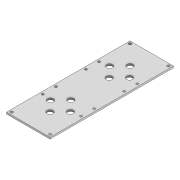
# Autodesk Inventor part: Cover
Saved by Autodesk Inventor 2022 (Build 260153000, 153)
## iProperties
Created: 2021-11-16
Part Number: Cover
Material: Generic
Document SubType Name: Modeling
Designer: Vking
Density: 1 g/cm^3
Appearance: Default
Author: Vking
Autodesk Inventor part; units mm, degrees
ref_plane "YZ Plane" through (0, 0, 0) normal (1, 0, 0) x (0, 1, 0)
ref_plane "XZ Plane" through (0, 0, 0) normal (0, 1, 0) x (-1, 0, 0)
ref_plane "XY Plane" through (0, 0, 0) normal (0, 0, 1) x (1, 0, 0)
sketch "Sketch1" plane through (0, 0, 0) normal (0, 1, 0) x (-1, 0, 0)
  line L0 (28.7334, 91.142) -> (-21.2666, 91.142)
  line L1 (-21.2666, 91.142) -> (-21.2666, -78.858)
  line L2 (-21.2666, -78.858) -> (28.7334, -78.858)
  line L3 (28.7334, -78.858) -> (28.7334, 91.142)
  line L4 (36.3534, 98.762) -> (-28.8866, 98.762)
  line L5 (-28.8866, 98.762) -> (-28.8866, -86.478)
  line L6 (-28.8866, -86.478) -> (36.3534, -86.478)
  line L7 (36.3534, -86.478) -> (36.3534, 98.762)
  circle A0 centre (3.7334, 66.142) radius 4.5
  circle A1 centre (18.7334, 50.521) radius 4.5
  circle A2 centre (3.7334, 34.892) radius 4.5
  circle A3 centre (-11.2666, 50.521) radius 4.5
  circle A4 centre (3.7334, -22.616) radius 4.5
  circle A5 centre (18.7334, -38.237) radius 4.5
  circle A6 centre (-11.2666, -38.237) radius 4.5
  circle A7 centre (3.7334, -53.858) radius 4.5
  circle A8 centre (32.5434, 94.952) radius 2
  circle A9 centre (-25.0766, 94.952) radius 2
  circle A10 centre (-25.0766, -82.668) radius 2
  circle A11 centre (32.5434, -82.668) radius 2
  circle A12 centre (32.3534, -16.3569) radius 1.695
  circle A13 centre (32.3656, 28.6431) radius 1.695
  circle A14 centre (32.3534, -36.0528) radius 1.6891
  circle A15 centre (32.3656, 48.339) radius 1.6891
  line L8 (3.7397, -95.1843) -> (3.7397, 116.3603) construction
  circle A16 centre (-24.874, -16.3569) radius 1.695
  circle A17 centre (-24.8862, 28.6431) radius 1.695
  circle A18 centre (-24.874, -36.0528) radius 1.6891
  circle A19 centre (-24.8862, 48.339) radius 1.6891
  point P0 (0, 0)
  dimension "d0" = 170
  dimension "d1" = 7.62
  dimension "d2" = 9
  dimension "d4" = 10
  dimension "d5" = 10
  dimension "d6" = 9
  dimension "d7" = 25
  dimension "d8" = 25
  dimension "d9" = 50
  dimension "d10" = 10
  dimension "d11" = 10
  dimension "d12" = 25
  dimension "d13" = 25
  dimension "d14" = 31.25
  dimension "d15" = 25
  dimension "d16" = 9
  dimension "d17" = 9
  dimension "d18" = 15.621
  dimension "d19" = 0
  dimension "d21" = 25
  dimension "d22" = 31.242
  dimension "d23" = 15.621
  dimension "d24" = 9
  dimension "d25" = 9
  dimension "d26" = 9
  dimension "d27" = 9
  dimension "d29" = 15.621
  dimension "d34" = 3.81
  dimension "d35" = 3.81
  dimension "d36" = 4
  dimension "d37" = 3.81
  dimension "d38" = 3.81
  dimension "d39" = 4
  dimension "d40" = 3.81
  dimension "d41" = 3.81
  dimension "d42" = 4
  dimension "d43" = 3.81
  dimension "d44" = 3.81
  dimension "d45" = 4
  dimension "d49" = 4
  dimension "d50" = 45
  dimension "d51" = 70.1211
  dimension "d52" = 3.9878
  dimension "d53" = 3.39
  dimension "d54" = 3.39
  dimension "d55" = 0
  dimension "d56" = 3.3782
  dimension "d57" = 0
  dimension "d58" = 23.08
  dimension "d59" = 23.08
  dimension "d60" = 32.6263
  dimension "d61" = 3.3782
  dimension "d62" = 4.0004
  constraints: 20 centre point, 18 end point, 4 parallel, 4 symmetric about line, 2 perpendicular, 1 horizontal, 1 vertical, 7 other
  measures "d0" distance of L2.end L0.start
  measures "d1" distance between parallel lines of L3 L7
  measures "d2" diameter of A1
  measures "d4" distance from line of A1.centre L3
  measures "d5" distance from line of L1 A3.centre
  measures "d6" diameter of A3
  measures "d7" distance from line of L1 A2.centre
  measures "d8" distance from line of L1 A0.centre
  measures "d9" distance of L1.end L2.end
  measures "d10" distance from line of L1 A6.centre
  measures "d11" distance from line of A5.centre L3
  measures "d12" distance from line of L1 A4.centre
  measures "d13" distance from line of L1 A7.centre
  measures "d14" distance of A2.centre A0.centre
  measures "d15" distance from line of L0 A0.centre
  measures "d16" diameter of A0
  measures "d17" diameter of A2
  measures "d18" vertical distance of A3.centre A0.centre
  measures "d19" vertical distance of A3.centre A1.centre
  measures "d21" distance from line of L2 A7.centre
  measures "d22" distance of A4.centre A7.centre
  measures "d23" vertical distance of A6.centre A4.centre
  measures "d24" diameter of A4
  measures "d25" diameter of A6
  measures "d26" diameter of A7
  measures "d27" diameter of A5
  measures "d29" vertical distance of A7.centre A5.centre
  measures "d34" distance from line of L6 A11.centre
  measures "d35" distance from line of A11.centre L7
  measures "d36" diameter of A11
  measures "d37" distance from line of L7 A8.centre
  measures "d38" distance from line of L4 A8.centre
  measures "d39" diameter of A8
  measures "d40" distance from line of L4 A9.centre
  measures "d41" distance from line of L5 A9.centre
  measures "d42" diameter of A9
  measures "d43" distance from line of L5 A10.centre
  measures "d44" distance from line of A10.centre L6
  measures "d45" diameter of A10
  measures "d49" distance from line of L7 A12.centre
  measures "d50" distance of A13.centre A12.centre
  measures "d51" distance from line of L6 A12.centre
  measures "d52" distance from line of L7 A13.centre
  measures "d53" diameter of A12
  measures "d54" diameter of A13
  measures "d55" horizontal distance of A12.centre A14.centre
  measures "d56" diameter of A15
  measures "d57" horizontal distance of A13.centre A15.centre
  measures "d60" distance between parallel lines of L8 L5
  measures "d61" diameter of A14
  measures "d62" distance from line of A19.centre L5
extrude "Extrusion1" add sketch "Sketch1" along normal blind 2.54 contours L3 L2 L1 L0 | L7 L6 L5 L4
body "Solid1"
